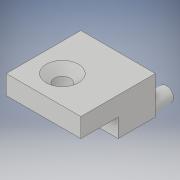
# Autodesk Inventor part: Door pin right
Saved by Autodesk Inventor 2019 (Build 230136000, 136)
## iProperties
Created: 2019-02-11
Part Number: Door pin right
Material: Generic
Document SubType Name: Modeling
Designer: aonih
Density: 1 g/cm^3
Appearance: Default
Author: aonih
Autodesk Inventor part; units mm, degrees
ref_plane "YZ Plane" through (0, 0, 0) normal (1, 0, 0) x (0, 1, 0)
ref_plane "XZ Plane" through (0, 0, 0) normal (0, 1, 0) x (-1, 0, 0)
ref_plane "XY Plane" through (0, 0, 0) normal (0, 0, 1) x (1, 0, 0)
sketch "Sketch2" plane through (0, 0, 0) normal (0, 1, 0) x (-1, 0, 0)
  line L0 (12.7, 12.7) -> (-12.7, 12.7)
  line L1 (-12.7, 12.7) -> (-12.7, -12.7)
  line L2 (-12.7, -12.7) -> (12.7, -12.7)
  line L3 (12.7, -12.7) -> (12.7, 12.7)
  line L4 (12.7, 0) -> (-12.7, 0) construction
  line L5 (0, -12.7) -> (0, 12.7) construction
  point P0 (0, 0)
  point P1 (0, 0)
  dimension "d2" = 25.4
  dimension "d3" = 25.4
  constraints: 12 end point, 5 midpoint, 2 parallel, 1 coincident, 1 horizontal, 1 perpendicular
  measures "d2" distance of L2.end L0.start
  measures "d3" distance of L1.end L2.end
extrude "Base" add sketch "Sketch2" against normal blind 6.5
sketch "Sketch10" plane through (0, -6.5, 0) normal (0, -1, 0) x (1, 0, 0)
  line L0 (-12.7, -12.7) -> (12.7, -12.7) projected
  line L1 (12.7, -12.7) -> (12.7, 0)
  line L2 (12.7, 0) -> (6.35, 0)
  line L3 (6.35, 0) -> (6.35, -12.7)
  line L4 (6.35, -12.7) -> (12.7, -12.7)
  line L5 (0, -12.7) -> (6.35, -12.7)
  line L6 (6.35, -12.7) -> (6.35, -6.35)
  line L7 (6.35, -6.35) -> (0, -6.35)
  line L8 (0, -6.35) -> (0, -12.7)
  point P0 (0, 0)
  dimension "d44" = 6.35
  dimension "d45" = 12.7
  dimension "d46" = 6.35
  dimension "d47" = 6.35
  constraints: 16 end point, 4 parallel, 3 perpendicular, 1 horizontal, 1 midpoint
  measures "d44" distance of L2.end L1.end
  measures "d45" distance of L0.end L1.end
  measures "d46" distance of L7.end L6.end
  measures "d47" distance of L6.end L5.end
extrude "Extrusion5" add sketch "Sketch10" along normal blind 6.35
sketch "Sketch11" plane through (0, 0, 0) normal (0, 1, 0) x (1, 0, 0)
  line L0 (12.7, -12.7) -> (-12.7, -12.7) projected
  line L1 (-12.7, -12.7) -> (-3.1541, -3.1541) construction
  line L2 (-12.7, -12.7) -> (0.8, -12.7) construction
  circle A0 centre (-3.1541, -3.1541) radius 5.5 construction
  point P0 (0, 0)
  dimension "d50" = 13.5
  dimension "d51" = 45
  dimension "d52" = 11
  constraints: 4 end point, 1 centre point, 1 coincident, 1 equal length, 1 horizontal
  measures "d50" distance of L0.end L1.end
  measures "d51" angle of L2 L1
  measures "d52" diameter of A0
hole "Hole3" at (-3.1541, 0, 3.1541) direction (0, -1, 0) diameter 5.5 end through all countersink diameter 11 countersink angle 90
sketch "Sketch12" plane through (12.7, 0, -12.7) normal (0, 0, -1) x (-1, 0, 0)
  line L0 (12.7, -6.5) -> (12.7, -12.85) projected
  line L1 (0, -6.5) -> (25.4, -6.5) construction
  line L2 (12.7, -6.5) -> (0, -6.5)
  line L3 (0, -6.5) -> (0, -12.85) construction
  line L4 (0, -12.85) -> (5, -12.85) construction
  line L5 (5, -12.85) -> (5, -7.85) construction
  line L6 (5, -7.85) -> (0, -7.85) construction
  line L7 (0, -7.85) -> (0, -12.85) construction
  line L8 (5, -7.85) -> (0, -12.85) construction
  line L9 (5, -12.85) -> (0, -7.85) construction
  circle A0 centre (2.5, -10.35) radius 2.425
  point P0 (12.7, 0)
  dimension "d60" = 5
  dimension "d61" = 5
  dimension "d62" = 4.85
  constraints: 14 end point, 2 parallel, 1 centre point, 1 collinear, 1 horizontal, 1 midpoint, 1 perpendicular
  measures "d60" distance of L6.end L5.end
  measures "d61" distance of L5.end L4.end
  measures "d62" diameter of A0
extrude "Extrusion6" add sketch "Sketch12" along normal blind 6.25
equation "\"d3\" = d2"
body "Solid1"
